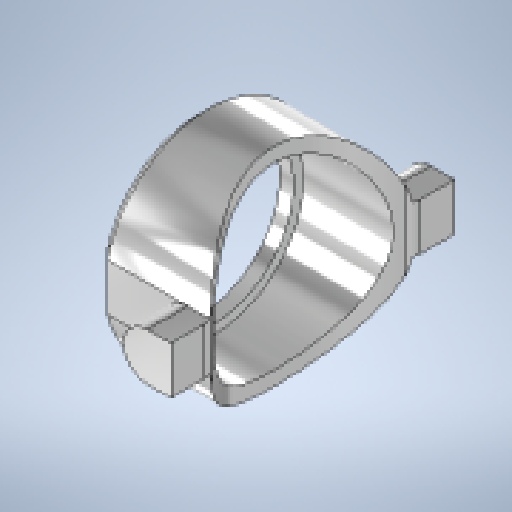
# Autodesk Inventor part: Cup
Saved by Autodesk Inventor 2023.2 (Build 272271000, 271)
## iProperties
Created: 2024-01-10
Part Number: Cup
Material: Aluminum 6061
Document SubType Name: Modeling
Designer: Nathan Cai
Density: 2.7 g/cm^3
Appearance: Aluminum - Flat
Mass: 3.40593 g
Surface Area: 17.3734 cm^2
Volume: 1.26146 cm^3
Author: Nathan Cai
Autodesk Inventor part; units mm, degrees
ref_plane "YZ Plane" through (0, 0, 0) normal (1, 0, 0) x (0, 1, 0)
ref_plane "XZ Plane" through (0, 0, 0) normal (0, 1, 0) x (-1, 0, 0)
ref_plane "XY Plane" through (0, 0, 0) normal (0, 0, 1) x (1, 0, 0)
sketch "Sketch1" plane through (0, 0, 0) normal (1, 0, 0) x (0, 1, 0)
  circle A0 centre (0, 0) radius 11
  circle A1 centre (0, 0) radius 8.5
  line L0 (2.5, 10.7121) -> (-2.5, 10.7121)
  line L1 (-2.5, 10.7121) -> (-2.5, -10.7121)
  line L2 (-2.5, -10.7121) -> (2.5, -10.7121)
  line L3 (2.5, -10.7121) -> (2.5, 10.7121)
  line L4 (2.5, 10.7121) -> (-2.5, -10.7121) construction
  line L5 (-2.5, 10.7121) -> (2.5, -10.7121) construction
  dimension "d0" = 22
  dimension "d3" = 17
  dimension "d18" = 5
  constraints: 12 end point, 2 coincident, 2 midpoint, 2 parallel, 1 centre point, 1 horizontal, 1 perpendicular, 3 other
  measures "d3" diameter of A1
  measures "d18" distance between parallel lines of L1 L3
extrude "Extrusion1" add sketch "Sketch1" along normal blind 12 contours A0 L3 A1 | L3 A1 L1 L0 | L2 L1 A1 L3 | L1 A1 A0
sketch "Sketch2" plane through (0, 0, 0) normal (0, 0, 1) x (1, 0, 0)
  line L0 (14.5, 2.5) -> (9.5, 2.5)
  line L1 (9.5, 2.5) -> (9.5, -2.5)
  line L2 (9.5, -2.5) -> (14.5, -2.5)
  line L3 (14.5, -2.5) -> (14.5, 2.5)
  line L4 (14.5, 2.5) -> (9.5, -2.5) construction
  line L5 (9.5, 2.5) -> (14.5, -2.5) construction
  circle A0 centre (9.5, 0) radius 2.5
  line L6 (12, -2.5) -> (12, 2.5) projected
  point P0 (0, 0)
  point P1 (12, 0)
  dimension "d4" = 5
  dimension "d5" = 5
  constraints: 12 end point, 4 midpoint, 2 parallel, 1 horizontal, 1 perpendicular, 3 other
  measures "d4" distance of L2.end L1.end
  measures "d5" distance of L1.end L0.end
extrude "Extrusion2" add sketch "Sketch2" along normal mid plane 30 contours L6 A0 L0 | A0 L1 | L1 A0 | L6 L2 A0
sketch "Sketch3" plane through (12, 0, 0) normal (1, 0, 0) x (0, 0, -1)
  circle A0 centre (0, 0) radius 9.5
  dimension "d8" = 19
  constraints: 1 centre point, 1 coincident
  measures "d8" diameter of A0
extrude "Extrusion3" cut sketch "Sketch3" against normal blind 10.5
chamfer "Chamfer1" distance 1 angle 45 4 edges at (0, -11, 0) (0, 11, 0) (0, 0, -10.7121) (0, 0, 10.7121)
sketch "Sketch4" plane through (0, 0, 0) normal (0, 1, 0) x (-1, 0, 0)
  line L0 (-12, 10.7121) -> (-12, -10.7121) projected
  circle A0 centre (-24, 0) radius 16.0857
  line L1 (-12, 0) -> (-24, 0) construction
  point P0 (0, 0)
  point P1 (-12, 10.7121)
  dimension "d14" = 12
  constraints: 2 end point, 1 horizontal, 1 midpoint, 3 other
  measures "d14" distance from line of L0 L1.end
extrude "Extrusion4" cut sketch "Sketch4" along normal through all both and the other way through all contours A0 L0 picked at (-10.6381, 0)
fillet "Fillet1" radius 2 2 edges at (12, 0, 10.7121) (12, 0, -10.7121)
equation "\"d1\" = Height"
equation "\"d9\" = Height - Flang_Thickness"
equation "\"Height\" = 12"
equation "\"Flang_Thickness\" = 1.5"
body "Solid1"
